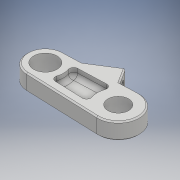
# Autodesk Inventor part: INVENTOR WORKSHOP
Saved by Autodesk Inventor 2017 (Build 210142000, 142)
## iProperties
Created: 2019-09-23
Part Number: INVENTOR WORKSHOP
Material: Generic
Document SubType Name: Modeling
Designer: Manan
Density: 1 g/cm^3
Appearance: Default
Author: Manan
Autodesk Inventor part; units mm, degrees
ref_plane "YZ Plane" through (0, 0, 0) normal (1, 0, 0) x (0, 1, 0)
ref_plane "XZ Plane" through (0, 0, 0) normal (0, 1, 0) x (-1, 0, 0)
ref_plane "XY Plane" through (0, 0, 0) normal (0, 0, 1) x (1, 0, 0)
sketch "Sketch1" plane through (0, 0, 0) normal (0, 0, 1) x (1, 0, 0)
  line L0 (-14, 0) -> (14, 0) construction
  line L1 (-14.25, 6.9955) -> (13.7143, 7.9949)
  line L2 (13.7143, -7.9949) -> (-14.25, -6.9955)
  arc A0 (-14.25, 6.9955) -> (-14.25, -6.9955) centre (-14, 0) ccw
  arc A1 (13.7143, -7.9949) -> (13.7143, 7.9949) centre (14, 0) ccw
  line L3 (-7.032, 7.2535) -> (3.1108, 13.6663)
  line L4 (3.1108, 13.6663) -> (6.8515, 7.7496)
  line L5 (4.9811, 10.708) -> (-0.0902, 7.5016) construction
  point P0 (0, 0)
  point P1 (0, 0)
  dimension "d0" = 8
  dimension "d1" = 7
  dimension "d2" = 28
  dimension "d3" = 12
  dimension "d4" = 7
  dimension "d5" = 3.5
  dimension "d6" = 14
  constraints: 14 end point, 4 point on circle, 4 tangent, 3 point on line, 2 centre point, 2 midpoint, 1 coincident, 1 horizontal, 1 parallel, 1 perpendicular
  measures "d0" radius of A1
  measures "d1" radius of A0
  measures "d2" distance of L0.start L0.end
  measures "d3" distance of L3.start L3.end
  measures "d4" distance of L3.end L4.end
  measures "d5" distance of L4.end L5.start
  measures "d6" distance of L0.end L5.start
extrude "Extrusion1" add sketch "Sketch1" along normal mid plane 6.35
hole "Hole1" at (14, 0, 3.175) direction (0, 0, -1) diameter 7.9375 end through all
hole "Hole2" at (-14, 0, 3.175) direction (0, 0, -1) diameter 9 end through all clearance for "Flat Head Machine Screw" size "M8" standard "Ansi Metric M Profile"
sketch "Sketch2" plane through (3.1108, 13.6663, 3.175) normal (0.8452325, 0.5343988, 0) x (0, 0, -1)
  point P0 (3.175, -9.8888)
sketch "Sketch3" plane through (3.1108, 13.6663, 3.175) normal (0.8452325, 0.5343988, 0) x (0, 0, -1)
  line L0 (0, -7) -> (0, 0) construction
  line L1 (0, -3.5) -> (6.35, -3.5) construction
  line L2 (6.35, 0) -> (6.35, -7) construction
  line L3 (6.35, 0) -> (0, 0) construction
  line L4 (3.175, 0) -> (3.175, -7) construction
  line L5 (6.35, -7) -> (0, -7) construction
  point P0 (3.175, -9.8888)
  point P1 (3.175, -3.5)
  constraints: 5 midpoint, 4 end point
hole "Hole3" at (4.9811, 10.708, 0) direction (-0.8452325, -0.5343988, 0) diameter 2.487 depth 5 tip angle 118 thread size "5-40 UNC" class "2B" standard "ANSI Unified Screw Threads"
sketch "Sketch4" plane through (0, 0, 3.175) normal (0, 0, 1) x (1, 0, 0)
  circle A0 centre (-14, 0) radius 4.5 projected
  circle A1 centre (14, 0) radius 3.9687 projected
  line L0 (6.8515, 7.7496) -> (3.1108, 13.6663) projected
  line L1 (3.1108, 13.6663) -> (-7.032, 7.2535) projected
  line L2 (-7.032, 7.2535) -> (-14.25, 6.9955) projected
  arc A2 (-14.25, 6.9955) -> (-14.25, -6.9955) centre (-14, 0) ccw projected
  line L3 (-14.25, -6.9955) -> (13.7143, -7.9949) projected
  arc A3 (13.7143, -7.9949) -> (13.7143, 7.9949) centre (14, 0) ccw projected
  line L4 (13.7143, 7.9949) -> (6.8515, 7.7496) projected
  line L5 (7.5804, -4.7738) -> (-8.402, -4.2026)
  arc A4 (-8.402, -4.2026) -> (-8.402, 4.2026) centre (-14, 0) ccw
  arc A5 (7.5804, 4.7738) -> (7.5804, -4.7738) centre (14, 0) ccw
  line L6 (-8.402, 4.2026) -> (7.5804, 4.7738)
  point P0 (0, 0)
  dimension "d35" = 3
  dimension "d36" = 3
  constraints: 6 end point, 5 point on circle, 2 centre point, 2 coincident, 2 concentric
  measures "d35" distance between parallel lines of L2 L6
  measures "d36" distance between parallel lines of L3 L5
extrude "Extrusion2" cut sketch "Sketch4" against normal blind 3.175 contours L5 A4 L6 A5
fillet "Fillet1" radius 1.5875 8 edges at (6, 0, 0) (7.5804, 4.7738, 1.5875) (-0.4108, 4.4882, 0) (-8.402, 4.2026, 1.5875) (-7, 0, 0) (-0.4108, -4.4882, 0) (7.5804, -4.7738, 1.5875) (-8.402, -4.2026, 1.5875)
chamfer "Chamfer1" distance 0.5 angle 45 14 edges at (-1.9606, 10.4599, -3.175) (-1.9606, 10.4599, 3.175) (-10.641, 7.1245, -3.175) (-21, 0, -3.175) (-0.2679, -7.4952, -3.175) (22, 0, -3.175) (10.2829, 7.8723, -3.175) (-10.641, 7.1245, 3.175) (-21, 0, 3.175) (-0.2679, -7.4952, 3.175) (22, 0, 3.175) (10.2829, 7.8723, 3.175) (4.9811, 10.708, -3.175) (4.9811, 10.708, 3.175)
fillet "Fillet2" radius 1 1 edges at (3.1108, 13.6663, 0)
fillet "Fillet3" radius 3.175 1 edges at (-7.032, 7.2535, 0)
body "Solid1"
